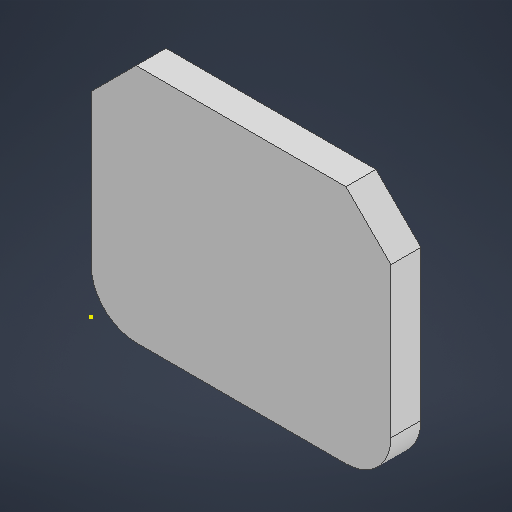
# Autodesk Inventor part: Part8
Saved by Autodesk Inventor 2026 (Build 300175050, 175E)
## iProperties
Created: 2026-03-19
Part Number: Part8
Material: Generic
Document SubType Name: Modeling
Designer: Administrator
Density: 1 g/cm^3
Appearance: Default
Author: Administrator
Autodesk Inventor part; units mm, degrees
ref_plane "YZ Plane" through (0, 0, 0) normal (1, 0, 0) x (0, 1, 0)
ref_plane "XZ Plane" through (0, 0, 0) normal (0, 1, 0) x (-1, 0, 0)
ref_plane "XY Plane" through (0, 0, 0) normal (0, 0, 1) x (1, 0, 0)
sketch "Sketch1" plane through (0, 0, 0) normal (0, 0, 1) x (1, 0, 0)
  line L0 (0, 0) -> (100, 0)
  line L1 (100, 0) -> (100, 80)
  line L2 (100, 80) -> (0, 80)
  line L3 (0, 80) -> (0, 0)
  circle A0 centre (15, 15) radius 5
  circle A1 centre (85, 15) radius 5
  circle A2 centre (85, 65) radius 5
  circle A3 centre (15, 65) radius 5
  dimension "d0" = 100
  dimension "d1" = 80
  dimension "d12" = 10
  dimension "d13" = 10
  dimension "d14" = 10
  dimension "d15" = 10
  dimension "d17" = 15
  dimension "d18" = 15
  dimension "d19" = 15
  dimension "d20" = 15
  dimension "d21" = 15
  dimension "d22" = 15
  dimension "d23" = 15
  dimension "d24" = 15
  constraints: 8 end point, 4 centre point, 3 perpendicular, 1 horizontal
  measures "d0" distance of L0.start L0.end
  measures "d1" distance of L2.end L0.start
  measures "d12" diameter of A2
  measures "d13" diameter of A1
  measures "d14" diameter of A3
  measures "d15" diameter of A0
  measures "d17" distance from line of L2 A3.centre
  measures "d18" distance from line of L3 A3.centre
  measures "d19" distance from line of L0 A0.centre
  measures "d20" distance from line of L3 A0.centre
  measures "d21" distance from line of L1 A1.centre
  measures "d22" distance from line of L0 A1.centre
  measures "d23" distance from line of L2 A2.centre
  measures "d24" distance from line of L1 A2.centre
extrude "Extrusion1" add sketch "Sketch1" along normal mid plane 10 contours L3 L2 L1 L0 | A0 | A1 | A2 | A3
sketch "Sketch2" plane through (0, 0, 5) normal (0, 0, 1) x (1, 0, 0)
  point P0 (0, 0)
chamfer "Chamfer1" distance 15 angle 45 1 edges at (100, 80, 0)
chamfer "Chamfer2" distance 15 angle 45 1 edges at (0, 80, 0)
fillet "Fillet1" radius 15 1 edges at (100, 0, 0)
fillet "Fillet2" radius 15 1 edges at (0, 0, 0)
sketch "Sketch3" plane through (0, 0, 5) normal (0, 0, 1) x (1, 0, 0)
  point P0 (0, 0)
body "Solid1"
